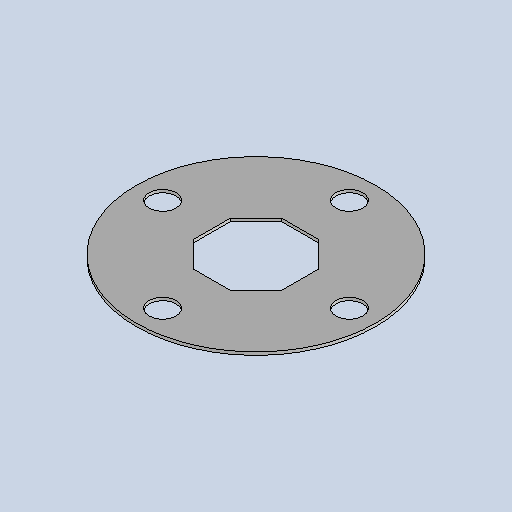
# Autodesk Inventor part: SLM 1792  funnel FLANGE 1200 50-90_1000x90
Saved by Autodesk Inventor 2025.3 (Build 293356030, 356C)
## iProperties
Created: 2025-06-24
Part Number: SLM 1792  funnel FLANGE 1200 50-90_1000x90
Material: Stainless Steel
Description: DIE16(5)|\ 90°|corrY -___°|X_____|bom___
Document SubType Name: Sheet Metal
Designer: user
Mass: 259.273 g
Surface Area: 342.578 cm^2
Volume: 32.4091 cm^3
Density: 8 g/cm^3
Flat Pattern Width: 16 cm
Flat Pattern Length: 16 cm
Flat Pattern Area: 256 cm^2
Sheet Metal Rule: Default
Sheet Metal Width: 160,000 mm
Sheet Metal Length: 160,000 mm
Sheet Metal Area: 25600,000 mm^2
Appearance: Default
Author: user
Autodesk Inventor part; units mm, degrees
ref_plane "YZ Plane" through (0, 0, 0) normal (1, 0, 0) x (0, 1, 0)
ref_plane "XZ Plane" through (0, 0, 0) normal (0, 1, 0) x (-1, 0, 0)
ref_plane "XY Plane" through (0, 0, 0) normal (0, 0, 1) x (1, 0, 0)
sketch "Sketch1" plane through (0, 0, 0) normal (0, 0, 1) x (1, 0, 0)
  circle A0 centre (0, 0) radius 62.5 construction
  circle A1 centre (0, 0) radius 29.5 construction
  circle A2 centre (0, 0) radius 80
  line L0 (12.2193, 29.5) -> (29.5, 12.2193)
  line L1 (29.5, 12.2193) -> (29.5, -12.2193)
  line L2 (29.5, -12.2193) -> (12.2193, -29.5)
  line L3 (12.2193, -29.5) -> (-12.2193, -29.5)
  line L4 (-12.2193, -29.5) -> (-29.5, -12.2193)
  line L5 (-29.5, -12.2193) -> (-29.5, 12.2193)
  line L6 (-29.5, 12.2193) -> (-12.2193, 29.5)
  line L7 (-12.2193, 29.5) -> (12.2193, 29.5)
  circle A3 centre (0, 62.5) radius 9
  circle A4 centre (-62.5, 0) radius 9
  circle A5 centre (0, -62.5) radius 9
  circle A6 centre (62.5, 0) radius 9
  point P0 (0, 29.5)
  dimension "D_b_c" = 125
  dimension "D_min" = 59
  dimension "D_max" = 160
  dimension "Blt_hl" = 18
  dimension "d177" = 360
  measures "D_max" diameter of A2
  measures "Blt_hl" diameter of A3
extrude "Plate5" add sketch "Sketch1" along normal blind 2
body "Solid3"
